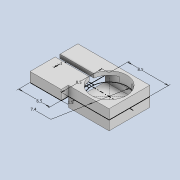
# Autodesk Inventor part: camera
Saved by Autodesk Inventor 2020 (Build 240168000, 168)
## iProperties
Created: 2020-08-31
Part Number: camera
Material: Generic
Document SubType Name: Modeling
Designer: songz
Density: 1 g/cm^3
Appearance: Default
Author: songz
Autodesk Inventor part; units mm, degrees
ref_plane "YZ Plane" through (0, 0, 0) normal (1, 0, 0) x (0, 1, 0)
ref_plane "XZ Plane" through (0, 0, 0) normal (0, 1, 0) x (-1, 0, 0)
ref_plane "XY Plane" through (0, 0, 0) normal (0, 0, 1) x (1, 0, 0)
sketch "Sketch1" plane through (0, 0, 0) normal (0, 1, 0) x (-1, 0, 0)
  line L0 (-4.25, -4.25) -> (4.25, -4.25)
  line L1 (4.25, -4.25) -> (4.25, 4.25)
  line L2 (4.25, 4.25) -> (-4.25, 4.25)
  line L3 (-4.25, 4.25) -> (-4.25, -4.25)
  line L4 (-4.25, -4.25) -> (4.25, 4.25) construction
  line L5 (4.25, -4.25) -> (-4.25, 4.25) construction
  circle A0 centre (0, 0) radius 3.7
  line L6 (10.75, 0.5) -> (3.6661, 0.5)
  line L7 (10.75, -0.5) -> (3.6661, -0.5)
  line L8 (6.6744, 0) -> (-5, 0)
  line L9 (4.25, 4.25) -> (4.25, 5.75)
  line L10 (4.25, 5.75) -> (10.75, 5.75)
  line L11 (10.75, 5.75) -> (10.75, -4.25)
  line L12 (10.75, -4.25) -> (4.25, -4.25)
  point P0 (4.25, 0.5)
  point P1 (4.25, -0.5)
  dimension "d0" = 8.5
  dimension "d1" = 8.5
  dimension "d2" = 7.4
  dimension "d6" = 1
  dimension "d9" = 1.5
  dimension "d10" = 6.5
  constraints: 26 end point, 6 point on line, 4 perpendicular, 3 horizontal, 3 parallel, 2 midpoint, 2 point on circle, 1 centre point, 1 coincident, 1 vertical, 1 other
  measures "d0" distance between parallel lines of L0 L2
  measures "d1" distance between parallel lines of L3 L1
  measures "d2" diameter of A0
  measures "d6" distance between parallel lines of L7 L6
  measures "d9" distance between parallel lines of L2 L10
  measures "d10" distance between parallel lines of L9 L11
extrude "Extrusion1" add sketch "Sketch1" along normal mid plane 4
shell "Shell2" thickness 0.8 removed faces 1 at (-10.75, 0.6667, 2.4167)
extrude "Extrusion2" cut sketch "Sketch1" along normal up to next contours L7 A0 L8 L1 | L1 L6 L11 L7 | L8 A0 | A0 L8 | L8 A0 L6 L1
extrude "Extrusion3" cut sketch "Sketch1" against normal up to next contours L1 L7 L11 L12 | L1 L6 L11 L7 | L9 L10 L11 L6 L1
body "Solid1"
